Autodesk Fusion 360 part; units mm, degrees
(part 2 of 4)
sketch "Sketch8" plane through (0, 0, 1.5) normal (0, 0, 1) x (-1, 0, 0)
  line L0 (-34.7574, -85.9106) -> (-28.1106, -92.5574)
  ellipse E0 centre (-28.8177, -93.2645) end of major axis (-25.9892, -96.0929) minor radius 1 (-29.5248, -93.9716) -> (-28.1106, -92.5574) ccw
  line L1 (-29.5248, -93.9716) -> (-36.1716, -87.3248)
  ellipse E1 centre (-35.4645, -86.6177) end of major axis (-32.636, -89.4461) minor radius 1 (-34.7574, -85.9106) -> (-36.1716, -87.3248) ccw
  ellipse E2 centre (-73.5355, -93.2645) end of major axis (-70.7071, -90.436) minor radius 1 (-74.2426, -92.5574) -> (-72.8284, -93.9716) ccw
  line L2 (-74.2426, -92.5574) -> (-56.8095, -75.1242)
  ellipse E3 centre (-56.1024, -75.8313) end of major axis (-53.2739, -73.0029) minor radius 1 (-55.3953, -76.5384) -> (-56.8095, -75.1242) ccw
  line L3 (-55.3953, -76.5384) -> (-72.8284, -93.9716)
  ellipse E4 centre (-38.4645, -75.7892) end of major axis (-35.636, -78.6177) minor radius 1 (-37.7574, -75.0821) -> (-39.1716, -76.4963) ccw
  line L4 (-37.7574, -75.0821) -> (-20.2821, -92.5574)
  ellipse E5 centre (-20.9892, -93.2645) end of major axis (-18.1608, -96.0929) minor radius 1 (-21.6963, -93.9716) -> (-20.2821, -92.5574) ccw
  line L5 (-21.6963, -93.9716) -> (-39.1716, -76.4963)
  ellipse E6 centre (-58.5355, -93.9213) end of major axis (-55.7071, -91.0929) minor radius 1 (-57.5048, -94.2952) -> (-58.9094, -92.8906) ccw
  ellipse E7 centre (-57.8787, -93.2645) end of major axis (-55.0503, -90.436) minor radius 1 (-58.9094, -92.8906) -> (-57.5048, -94.2952) ccw
  ellipse E8 centre (-65.7071, -93.2645) end of major axis (-62.8787, -90.436) minor radius 1 (-66.4142, -92.5574) -> (-65, -93.9716) ccw
  line L6 (-66.4142, -92.5574) -> (-59.2426, -85.3858)
  ellipse E9 centre (-58.5355, -86.0929) end of major axis (-55.7071, -83.2645) minor radius 1 (-57.8284, -86.8) -> (-59.2426, -85.3858) ccw
  line L7 (-57.8284, -86.8) -> (-65, -93.9716)
  ellipse E10 centre (-35.6289, -93.7569) end of major axis (-32.8005, -96.5853) minor radius 1 (-35.1707, -92.8062) -> (-36.5796, -94.2151) ccw
  ellipse E11 centre (-36.1213, -93.2645) end of major axis (-33.2929, -96.0929) minor radius 1 (-36.5796, -94.2151) -> (-35.1707, -92.8062) ccw
  line L8 (-93.75, -111.8) -> (-0.25, -111.8)
  line L9 (-0.25, -111.8) -> (-0.25, -0.25)
  line L10 (-0.25, -0.25) -> (-93.75, -0.25)
  line L11 (-93.75, -0.25) -> (-93.75, -111.8)
  circle A0 centre (-5, -5) radius 2
  circle A1 centre (-3.5, -95.55) radius 2
  circle A2 centre (-90.5, -95.55) radius 2
  circle A3 centre (-87.5, -6.5) radius 2
  line L12 (-42.5, -83.8) -> (-42.5, -96.8)
  line L13 (-42.5, -96.8) -> (-51.5, -96.8)
  line L14 (-51.5, -96.8) -> (-51.5, -83.8)
  line L15 (-51.5, -83.8) -> (-42.5, -83.8)
  line L16 (-42, -100.3) -> (-42, -110.3)
  line L17 (-42, -110.3) -> (-43.9689, -110.3)
  line L18 (-43.9689, -110.3) -> (-43.9689, -103.55)
  line L19 (-43.9689, -103.55) -> (-47, -101.8)
  line L20 (-47, -101.8) -> (-50.0311, -103.55)
  line L21 (-50.0311, -103.55) -> (-50.0311, -110.3)
  line L22 (-50.0311, -110.3) -> (-52, -110.3)
  line L23 (-52, -110.3) -> (-52, -100.3)
  line L24 (-52, -100.3) -> (-55, -100.3)
  line L25 (-55, -100.3) -> (-55, -80.3)
  line L26 (-55, -80.3) -> (-52, -80.3)
  line L27 (-52, -80.3) -> (-52, -81.8)
  line L28 (-52, -81.8) -> (-53.5, -81.8)
  line L29 (-53.5, -81.8) -> (-53.5, -98.8)
  line L30 (-53.5, -98.8) -> (-40.5, -98.8)
  line L31 (-40.5, -98.8) -> (-40.5, -81.8)
  line L32 (-40.5, -81.8) -> (-42, -81.8)
  line L33 (-42, -81.8) -> (-42, -80.3)
  line L34 (-42, -80.3) -> (-39, -80.3)
  line L35 (-39, -80.3) -> (-39, -100.3)
  line L36 (-39, -100.3) -> (-42, -100.3)
  line L37 (-0.25, -111.8) -> (-15.25, -111.8)
  line L38 (-15.25, -111.8) -> (-15.25, -96.8)
  line L39 (-15.25, -96.8) -> (-0.25, -96.8)
  line L40 (-0.25, -96.8) -> (-0.25, -111.8)
  line L41 (-93.75, -0.25) -> (-78.75, -0.25)
  line L42 (-78.75, -0.25) -> (-78.75, -15.25)
  line L43 (-78.75, -15.25) -> (-93.75, -15.25)
  line L44 (-93.75, -15.25) -> (-93.75, -0.25)
  line L45 (-78.75, -15.25) -> (-15.25, -15.25)
  line L46 (-15.25, -15.25) -> (-15.25, -96.8)
  line L47 (-15.25, -96.8) -> (-78.75, -96.8)
  line L48 (-78.75, -96.8) -> (-78.75, -15.25)
  line L49 (-47, -96.8) -> (-42, -96.8)
  line L50 (-42, -96.8) -> (-42, -15.25)
  line L51 (-42, -15.25) -> (-47, -15.25)
  line L52 (-47, -15.25) -> (-47, -96.8)
  line L53 (-47, -15.25) -> (-52, -15.25)
  line L54 (-52, -15.25) -> (-52, -96.8)
  line L55 (-52, -96.8) -> (-47, -96.8)
  line L56 (-47, -96.8) -> (-47, -15.25)
  line L57 (-52, -15.25) -> (-78.75, -15.25)
  line L58 (-78.75, -15.25) -> (-78.75, -17.25)
  line L59 (-78.75, -17.25) -> (-52, -17.25)
  line L60 (-52, -17.25) -> (-52, -15.25)
  line L61 (-52, -17.25) -> (-78.75, -17.25)
  line L62 (-78.75, -17.25) -> (-78.75, -22.25)
  line L63 (-78.75, -22.25) -> (-52, -22.25)
  line L64 (-52, -22.25) -> (-52, -17.25)
  line L65 (-52, -17.25) -> (-56, -17.25)
  line L66 (-56, -17.25) -> (-56, -15.25)
  line L67 (-56, -15.25) -> (-52, -15.25)
  line L68 (-52, -15.25) -> (-52, -17.25)
  line L69 (-78.75, -17.25) -> (-74.75, -17.25)
  line L70 (-74.75, -17.25) -> (-74.75, -15.25)
  line L71 (-74.75, -15.25) -> (-78.75, -15.25)
  line L72 (-78.75, -15.25) -> (-78.75, -17.25)
  ellipse E12 centre (-56, -16.25) end of major axis (-56, -17.25) minor radius 4
  line L73 (-56, -15.25) -> (-56, -17.25)
  line L74 (-60, -16.25) -> (-52, -16.25)
  ellipse E13 centre (-74.75, -16.25) end of major axis (-74.75, -17.25) minor radius 4
  line L75 (-74.75, -15.25) -> (-74.75, -17.25)
  line L76 (-78.75, -16.25) -> (-70.75, -16.25)
  line L77 (-52, -22.25) -> (-78.75, -22.25)
  ellipse E14 centre (-74.75, -23.25) end of major axis (-74.75, -24.25) minor radius 4
  line L78 (-74.75, -22.25) -> (-74.75, -24.25)
  line L79 (-78.75, -23.25) -> (-70.75, -23.25)
  line L80 (-52, -24.25) -> (-52, -22.25)
  line L81 (-78.75, -22.25) -> (-78.75, -24.25)
  line L82 (-52, -24.25) -> (-56, -24.25)
  line L83 (-52, -22.25) -> (-52, -24.25)
  line L84 (-56, -22.25) -> (-56, -24.25) construction
  line L85 (-60, -23.25) -> (-52, -23.25) construction
  line L86 (-74.75, -22.25) -> (-78.75, -22.25)
  line L87 (-78.75, -24.25) -> (-78.75, -29.25)
  line L88 (-78.75, -22.25) -> (-78.75, -24.25)
  ellipse E15 centre (-56, -23.25) end of major axis (-56, -24.25) minor radius 4
  line L89 (-56, -22.25) -> (-56, -24.25)
  line L90 (-60, -23.25) -> (-52, -23.25)
  line L91 (-74.75, -24.25) -> (-74.75, -22.25)
  line L92 (-56, -22.25) -> (-52, -22.25)
  line L93 (-52, -29.25) -> (-52, -24.25)
  line L94 (-78.75, -24.25) -> (-74.75, -24.25)
  line L95 (-78.75, -24.25) -> (-52, -24.25)
  line L96 (-52, -24.25) -> (-78.75, -24.25)
  line L97 (-56, -24.25) -> (-56, -22.25)
  line L98 (-78.75, -29.25) -> (-52, -29.25)
  line L99 (-52, -29.25) -> (-78.75, -29.25)
  line L100 (-78.75, -31.25) -> (-52, -31.25)
  line L101 (-78.75, -38.25) -> (-52, -38.25)
  line L102 (-52, -36.25) -> (-78.75, -36.25)
  line L103 (-78.75, -43.25) -> (-52, -43.25)
  line L104 (-78.75, -36.25) -> (-52, -36.25)
  line L105 (-56, -36.25) -> (-56, -38.25) construction
  line L106 (-52, -31.25) -> (-78.75, -31.25)
  line L107 (-52, -38.25) -> (-78.75, -38.25)
  line L108 (-74.75, -29.25) -> (-78.75, -29.25)
  line L109 (-56, -36.25) -> (-52, -36.25)
  line L110 (-52, -36.25) -> (-52, -38.25)
  line L111 (-56, -29.25) -> (-56, -31.25) construction
  line L112 (-52, -38.25) -> (-52, -36.25)
  line L113 (-60, -30.25) -> (-52, -30.25) construction
  line L114 (-60, -37.25) -> (-52, -37.25) construction
  ellipse E16 centre (-56, -37.25) end of major axis (-56, -38.25) minor radius 4
  line L115 (-56, -36.25) -> (-56, -38.25)
  line L116 (-60, -37.25) -> (-52, -37.25)
  ellipse E17 centre (-74.75, -37.25) end of major axis (-74.75, -38.25) minor radius 4
  line L117 (-74.75, -36.25) -> (-74.75, -38.25)
  line L118 (-78.75, -37.25) -> (-70.75, -37.25)
  line L119 (-52, -43.25) -> (-52, -38.25)
  line L120 (-56, -36.25) -> (-56, -38.25) construction
  line L121 (-78.75, -38.25) -> (-78.75, -43.25)
  line L122 (-52, -31.25) -> (-56, -31.25)
  line L123 (-74.75, -36.25) -> (-78.75, -36.25)
  line L124 (-78.75, -29.25) -> (-78.75, -31.25)
  line L125 (-78.75, -38.25) -> (-74.75, -38.25)
  line L126 (-78.75, -36.25) -> (-78.75, -38.25)
  line L127 (-56, -29.25) -> (-52, -29.25)
  line L128 (-78.75, -31.25) -> (-78.75, -36.25)
  line L129 (-74.75, -38.25) -> (-74.75, -36.25)
  line L130 (-52, -29.25) -> (-52, -31.25)
  line L131 (-78.75, -36.25) -> (-78.75, -38.25)
  line L132 (-56, -31.25) -> (-56, -29.25)
  line L133 (-56, -38.25) -> (-56, -36.25)
  line L134 (-78.75, -29.25) -> (-78.75, -31.25)
  line L135 (-60, -37.25) -> (-52, -37.25) construction
  line L136 (-78.75, -31.25) -> (-74.75, -31.25)
  line L137 (-52, -38.25) -> (-56, -38.25)
  ellipse E18 centre (-56, -30.25) end of major axis (-56, -31.25) minor radius 4
  line L138 (-56, -29.25) -> (-56, -31.25)
  line L139 (-60, -30.25) -> (-52, -30.25)
  line L140 (-74.75, -31.25) -> (-74.75, -29.25)
  line L141 (-52, -36.25) -> (-52, -31.25)
  ellipse E19 centre (-74.75, -30.25) end of major axis (-74.75, -31.25) minor radius 4
  line L142 (-74.75, -29.25) -> (-74.75, -31.25)
  line L143 (-78.75, -30.25) -> (-70.75, -30.25)
  line L144 (-52, -31.25) -> (-52, -29.25)
  line L145 (-78.75, -66.25) -> (-52, -66.25)
  line L146 (-52, -52.25) -> (-78.75, -52.25)
  line L147 (-78.75, -58.25) -> (-70.75, -58.25) construction
  line L148 (-56, -52.25) -> (-56, -50.25)
  ellipse E20 centre (-74.75, -58.25) end of major axis (-74.75, -59.25) minor radius 4
  line L149 (-74.75, -57.25) -> (-74.75, -59.25)
  line L150 (-78.75, -58.25) -> (-70.75, -58.25)
  line L151 (-78.75, -51.25) -> (-70.75, -51.25) construction
  line L152 (-56, -50.25) -> (-56, -52.25) construction
  ellipse E21 centre (-74.75, -44.25) end of major axis (-74.75, -45.25) minor radius 4
  line L153 (-74.75, -43.25) -> (-74.75, -45.25)
  line L154 (-78.75, -44.25) -> (-70.75, -44.25)
  line L155 (-60, -58.25) -> (-52, -58.25) construction
  line L156 (-56, -43.25) -> (-56, -45.25) construction
  line L157 (-78.75, -66.25) -> (-74.75, -66.25)
  line L158 (-56, -64.25) -> (-56, -66.25) construction
  line L159 (-52, -43.25) -> (-52, -45.25)
  line L160 (-60, -44.25) -> (-52, -44.25) construction
  ellipse E22 centre (-56, -58.25) end of major axis (-56, -59.25) minor radius 4
  line L161 (-56, -57.25) -> (-56, -59.25)
  line L162 (-60, -58.25) -> (-52, -58.25)
  line L163 (-52, -52.25) -> (-52, -50.25)
  line L164 (-56, -66.25) -> (-56, -64.25)
  line L165 (-56, -57.25) -> (-56, -59.25) construction
  ellipse E23 centre (-56, -44.25) end of major axis (-56, -45.25) minor radius 4
  line L166 (-56, -43.25) -> (-56, -45.25)
  line L167 (-60, -44.25) -> (-52, -44.25)
  ellipse E24 centre (-74.75, -51.25) end of major axis (-74.75, -52.25) minor radius 4
  line L168 (-74.75, -50.25) -> (-74.75, -52.25)
  line L169 (-78.75, -51.25) -> (-70.75, -51.25)
  line L170 (-74.75, -64.25) -> (-78.75, -64.25)
  line L171 (-78.75, -57.25) -> (-78.75, -59.25)
  line L172 (-78.75, -50.25) -> (-78.75, -52.25)
  line L173 (-74.75, -50.25) -> (-78.75, -50.25)
  line L174 (-74.75, -59.25) -> (-74.75, -57.25)
  line L175 (-52, -43.25) -> (-78.75, -43.25)
  line L176 (-78.75, -43.25) -> (-78.75, -45.25)
  line L177 (-60, -65.25) -> (-52, -65.25) construction
  line L178 (-52, -64.25) -> (-52, -66.25)
  line L179 (-78.75, -64.25) -> (-78.75, -66.25)
  line L180 (-56, -64.25) -> (-56, -66.25) construction
  line L181 (-74.75, -57.25) -> (-78.75, -57.25)
  line L182 (-78.75, -65.25) -> (-70.75, -65.25) construction
  line L183 (-74.75, -43.25) -> (-78.75, -43.25)
  line L184 (-52, -66.25) -> (-52, -64.25)
  line L185 (-56, -64.25) -> (-56, -66.25) construction
  line L186 (-74.75, -64.25) -> (-74.75, -66.25) construction
  line L187 (-74.75, -52.25) -> (-74.75, -50.25)
  line L188 (-74.75, -45.25) -> (-74.75, -43.25)
  line L189 (-78.75, -59.25) -> (-78.75, -64.25)
  line L190 (-52, -59.25) -> (-52, -57.25)
  line L191 (-78.75, -52.25) -> (-74.75, -52.25)
  line L192 (-78.75, -50.25) -> (-78.75, -52.25)
  line L193 (-60, -65.25) -> (-52, -65.25) construction
  line L194 (-56, -64.25) -> (-52, -64.25)
  ellipse E25 centre (-74.75, -65.25) end of major axis (-74.75, -66.25) minor radius 4
  line L195 (-74.75, -64.25) -> (-74.75, -66.25)
  line L196 (-78.75, -65.25) -> (-70.75, -65.25)
  line L197 (-78.75, -57.25) -> (-78.75, -59.25)
  line L198 (-52, -64.25) -> (-52, -59.25)
  line L199 (-78.75, -59.25) -> (-52, -59.25)
  line L200 (-56, -59.25) -> (-56, -57.25)
  line L201 (-56, -50.25) -> (-56, -52.25) construction
  line L202 (-56, -43.25) -> (-52, -43.25)
  line L203 (-60, -51.25) -> (-52, -51.25) construction
  ellipse E26 centre (-56, -51.25) end of major axis (-56, -52.25) minor radius 4
  line L204 (-56, -50.25) -> (-56, -52.25)
  line L205 (-60, -51.25) -> (-52, -51.25)
  line L206 (-56, -50.25) -> (-52, -50.25)
  line L207 (-78.75, -45.25) -> (-52, -45.25)
  line L208 (-56, -45.25) -> (-56, -43.25)
  line L209 (-52, -59.25) -> (-78.75, -59.25)
  line L210 (-78.75, -57.25) -> (-52, -57.25)
  line L211 (-78.75, -71.25) -> (-52, -71.25)
  line L212 (-78.75, -64.25) -> (-52, -64.25)
  line L213 (-52, -64.25) -> (-78.75, -64.25)
  line L214 (-52, -66.25) -> (-78.75, -66.25)
  line L215 (-78.75, -52.25) -> (-52, -52.25)
  line L216 (-60, -51.25) -> (-52, -51.25) construction
  line L217 (-78.75, -52.25) -> (-78.75, -57.25)
  line L218 (-74.75, -66.25) -> (-74.75, -64.25)
  line L219 (-56, -57.25) -> (-52, -57.25)
  line L220 (-78.75, -50.25) -> (-52, -50.25)
  line L221 (-52, -57.25) -> (-52, -52.25)
  line L222 (-52, -57.25) -> (-78.75, -57.25)
  line L223 (-52, -50.25) -> (-78.75, -50.25)
  line L224 (-52, -52.25) -> (-56, -52.25)
  line L225 (-52, -45.25) -> (-78.75, -45.25)
  line L226 (-47, -43.25) -> (-52, -43.25)
  line L227 (-78.75, -59.25) -> (-74.75, -59.25)
  line L228 (-78.75, -43.25) -> (-78.75, -45.25)
  line L229 (-78.75, -66.25) -> (-78.75, -71.25)
  line L230 (-78.75, -45.25) -> (-78.75, -50.25)
  line L231 (-60, -65.25) -> (-52, -65.25) construction
  line L232 (-52, -71.25) -> (-52, -66.25)
  ellipse E27 centre (-56, -65.25) end of major axis (-56, -66.25) minor radius 4
  line L233 (-56, -64.25) -> (-56, -66.25)
  line L234 (-60, -65.25) -> (-52, -65.25)
  line L235 (-52, -59.25) -> (-56, -59.25)
  line L236 (-78.75, -45.25) -> (-74.75, -45.25)
  line L237 (-52, -57.25) -> (-52, -59.25)
  line L238 (-78.75, -64.25) -> (-78.75, -66.25)
  line L239 (-52, -66.25) -> (-56, -66.25)
  line L240 (-52, -45.25) -> (-56, -45.25)
  line L241 (-52, -50.25) -> (-52, -45.25)
  line L242 (-52, -45.25) -> (-52, -43.25)
  line L243 (-52, -50.25) -> (-52, -52.25)
  line L244 (-15.25, -57.25) -> (-15.25, -52.25)
  line L245 (-15.25, -24.25) -> (-42, -24.25)
  line L246 (-42, -59.25) -> (-15.25, -59.25)
  line L247 (-15.25, -66.25) -> (-42, -66.25)
  line L248 (-42, -57.25) -> (-15.25, -57.25)
  line L249 (-15.25, -64.25) -> (-42, -64.25)
  ellipse E28 centre (-19.25, -44.25) end of major axis (-19.25, -45.25) minor radius 4
  line L250 (-19.25, -43.25) -> (-19.25, -45.25)
  line L251 (-23.25, -44.25) -> (-15.25, -44.25)
  line L252 (-42, -45.25) -> (-15.25, -45.25)
  line L253 (-15.25, -50.25) -> (-42, -50.25)
  line L254 (-15.25, -36.25) -> (-42, -36.25)
  line L255 (-15.25, -52.25) -> (-42, -52.25)
  line L256 (-42, -24.25) -> (-15.25, -24.25)
  line L257 (-23.25, -51.25) -> (-15.25, -51.25) construction
  line L258 (-15.25, -29.25) -> (-42, -29.25)
  line L259 (-15.25, -38.25) -> (-42, -38.25)
  line L260 (-15.25, -64.25) -> (-15.25, -66.25)
  line L261 (-19.25, -66.25) -> (-19.25, -64.25)
  line L262 (-19.25, -43.25) -> (-15.25, -43.25)
  line L263 (-42, -22.25) -> (-15.25, -22.25)
  line L264 (-42, -29.25) -> (-15.25, -29.25)
  line L265 (-42, -59.25) -> (-42, -64.25)
  line L266 (-19.25, -50.25) -> (-15.25, -50.25)
  ellipse E29 centre (-19.25, -58.25) end of major axis (-19.25, -59.25) minor radius 4
  line L267 (-19.25, -57.25) -> (-19.25, -59.25)
  line L268 (-23.25, -58.25) -> (-15.25, -58.25)
  ellipse E30 centre (-19.25, -65.25) end of major axis (-19.25, -66.25) minor radius 4
  line L269 (-19.25, -64.25) -> (-19.25, -66.25)
  line L270 (-23.25, -65.25) -> (-15.25, -65.25)
  line L271 (-15.25, -59.25) -> (-19.25, -59.25)
  line L272 (-19.25, -50.25) -> (-19.25, -52.25) construction
  line L273 (-19.25, -15.25) -> (-19.25, -17.25) construction
  line L274 (-42, -38.25) -> (-42, -43.25)
  line L275 (-38, -24.25) -> (-38, -22.25)
  line L276 (-42, -65.25) -> (-34, -65.25) construction
  line L277 (-19.25, -24.25) -> (-19.25, -22.25)
  line L278 (-15.25, -38.25) -> (-19.25, -38.25)
  line L279 (-15.25, -22.25) -> (-15.25, -24.25)
  line L280 (-15.25, -29.25) -> (-15.25, -31.25)
  line L281 (-42, -58.25) -> (-34, -58.25) construction
  line L282 (-23.25, -30.25) -> (-15.25, -30.25) construction
  line L283 (-15.25, -24.25) -> (-19.25, -24.25)
  line L284 (-23.25, -37.25) -> (-15.25, -37.25) construction
  line L285 (-23.25, -51.25) -> (-15.25, -51.25) construction
  line L286 (-23.25, -16.25) -> (-15.25, -16.25) construction
  line L287 (-15.25, -50.25) -> (-15.25, -45.25)
  line L288 (-15.25, -31.25) -> (-15.25, -29.25)
  line L289 (-19.25, -36.25) -> (-15.25, -36.25)
  line L290 (-42, -24.25) -> (-38, -24.25)
  line L291 (-42, -31.25) -> (-38, -31.25)
  line L292 (-15.25, -38.25) -> (-15.25, -36.25)
  line L293 (-38, -59.25) -> (-38, -57.25)
  line L294 (-19.25, -29.25) -> (-19.25, -31.25) construction
  line L295 (-19.25, -50.25) -> (-19.25, -52.25) construction
  line L296 (-19.25, -36.25) -> (-19.25, -38.25) construction
  line L297 (-23.25, -23.25) -> (-15.25, -23.25) construction
  line L298 (-42, -44.25) -> (-34, -44.25) construction
  line L299 (-42, -16.25) -> (-34, -16.25) construction
  ellipse E31 centre (-19.25, -16.25) end of major axis (-19.25, -17.25) minor radius 4
  line L300 (-19.25, -15.25) -> (-19.25, -17.25)
  line L301 (-23.25, -16.25) -> (-15.25, -16.25)
  line L302 (-42, -15.25) -> (-42, -17.25)
  line L303 (-19.25, -31.25) -> (-19.25, -29.25)
  line L304 (-19.25, -45.25) -> (-19.25, -43.25)
  line L305 (-38, -22.25) -> (-42, -22.25)
  line L306 (-42, -22.25) -> (-42, -24.25)
  line L307 (-15.25, -45.25) -> (-15.25, -43.25)
  ellipse E32 centre (-38, -65.25) end of major axis (-38, -66.25) minor radius 4
  line L308 (-38, -64.25) -> (-38, -66.25)
  line L309 (-42, -65.25) -> (-34, -65.25)
  line L310 (-19.25, -36.25) -> (-19.25, -38.25) construction
  line L311 (-42, -58.25) -> (-34, -58.25) construction
  line L312 (-19.25, -50.25) -> (-19.25, -52.25) construction
  ellipse E33 centre (-38, -58.25) end of major axis (-38, -59.25) minor radius 4
  line L313 (-38, -57.25) -> (-38, -59.25)
  line L314 (-42, -58.25) -> (-34, -58.25)
  line L315 (-38, -64.25) -> (-38, -66.25) construction
  line L316 (-42, -51.25) -> (-34, -51.25) construction
  line L317 (-19.25, -15.25) -> (-15.25, -15.25)
  line L318 (-23.25, -51.25) -> (-15.25, -51.25) construction
  line L319 (-42, -15.25) -> (-42, -17.25)
  line L320 (-19.25, -38.25) -> (-19.25, -36.25)
  line L321 (-38, -22.25) -> (-38, -24.25) construction
  line L322 (-42, -22.25) -> (-42, -24.25)
  line L323 (-19.25, -17.25) -> (-19.25, -15.25)
  line L324 (-15.25, -52.25) -> (-19.25, -52.25)
  line L325 (-19.25, -29.25) -> (-15.25, -29.25)
  ellipse E34 centre (-19.25, -51.25) end of major axis (-19.25, -52.25) minor radius 4
  line L326 (-19.25, -50.25) -> (-19.25, -52.25)
  line L327 (-23.25, -51.25) -> (-15.25, -51.25)
  line L328 (-23.25, -58.25) -> (-15.25, -58.25) construction
  line L329 (-15.25, -45.25) -> (-42, -45.25)
  line L330 (-42, -31.25) -> (-42, -36.25)
  ellipse E35 centre (-38, -51.25) end of major axis (-38, -52.25) minor radius 4
  line L331 (-38, -50.25) -> (-38, -52.25)
  line L332 (-42, -51.25) -> (-34, -51.25)
  line L333 (-38, -52.25) -> (-38, -50.25)
  line L334 (-42, -45.25) -> (-42, -50.25)
  line L335 (-38, -31.25) -> (-38, -29.25)
  line L336 (-42, -52.25) -> (-38, -52.25)
  ellipse E36 centre (-38, -37.25) end of major axis (-38, -38.25) minor radius 4
  line L337 (-38, -36.25) -> (-38, -38.25)
  line L338 (-42, -37.25) -> (-34, -37.25)
  line L339 (-42, -50.25) -> (-42, -52.25)
  line L340 (-42, -38.25) -> (-38, -38.25)
  line L341 (-42, -30.25) -> (-34, -30.25) construction
  line L342 (-42, -36.25) -> (-42, -38.25)
  ellipse E37 centre (-38, -44.25) end of major axis (-38, -45.25) minor radius 4
  line L343 (-38, -43.25) -> (-38, -45.25)
  line L344 (-42, -44.25) -> (-34, -44.25)
  line L345 (-42, -43.25) -> (-42, -45.25)
  line L346 (-38, -50.25) -> (-42, -50.25)
  line L347 (-38, -43.25) -> (-42, -43.25)
  line L348 (-42, -29.25) -> (-42, -31.25)
  line L349 (-38, -38.25) -> (-38, -36.25)
  line L350 (-23.25, -23.25) -> (-15.25, -23.25) construction
  ellipse E38 centre (-38, -30.25) end of major axis (-38, -31.25) minor radius 4
  line L351 (-38, -29.25) -> (-38, -31.25)
  line L352 (-42, -30.25) -> (-34, -30.25)
  line L353 (-19.25, -22.25) -> (-15.25, -22.25)
  line L354 (-10.25, -43.25) -> (-15.25, -43.25)
  line L355 (-15.25, -36.25) -> (-15.25, -38.25)
  line L356 (-42, -50.25) -> (-42, -52.25)
  line L357 (-38, -15.25) -> (-38, -17.25) construction
  line L358 (-19.25, -29.25) -> (-19.25, -31.25) construction
  line L359 (-15.25, -31.25) -> (-19.25, -31.25)
  line L360 (-15.25, -36.25) -> (-15.25, -31.25)
  line L361 (-42, -23.25) -> (-34, -23.25) construction
  line L362 (-23.25, -37.25) -> (-15.25, -37.25) construction
  line L363 (-38, -36.25) -> (-42, -36.25)
  line L364 (-15.25, -22.25) -> (-15.25, -17.25)
  line L365 (-38, -45.25) -> (-38, -43.25)
  ellipse E39 centre (-19.25, -30.25) end of major axis (-19.25, -31.25) minor radius 4
  line L366 (-19.25, -29.25) -> (-19.25, -31.25)
  line L367 (-23.25, -30.25) -> (-15.25, -30.25)
  line L368 (-42, -36.25) -> (-42, -38.25)
  line L369 (-15.25, -43.25) -> (-15.25, -45.25)
  line L370 (-38, -17.25) -> (-38, -15.25)
  line L371 (-23.25, -37.25) -> (-15.25, -37.25) construction
  line L372 (-19.25, -22.25) -> (-19.25, -24.25) construction
  line L373 (-19.25, -22.25) -> (-19.25, -24.25) construction
  line L374 (-15.25, -24.25) -> (-15.25, -22.25)
  line L375 (-23.25, -30.25) -> (-15.25, -30.25) construction
  ellipse E40 centre (-38, -16.25) end of major axis (-38, -17.25) minor radius 4
  line L376 (-38, -15.25) -> (-38, -17.25)
  line L377 (-42, -16.25) -> (-34, -16.25)
  line L378 (-38, -15.25) -> (-42, -15.25)
  line L379 (-38, -29.25) -> (-42, -29.25)
  ellipse E41 centre (-38, -23.25) end of major axis (-38, -24.25) minor radius 4
  line L380 (-38, -22.25) -> (-38, -24.25)
  line L381 (-42, -23.25) -> (-34, -23.25)
  line L382 (-15.25, -15.25) -> (-15.25, -17.25)
  line L383 (-42, -43.25) -> (-42, -45.25)
  ellipse E42 centre (-19.25, -37.25) end of major axis (-19.25, -38.25) minor radius 4
  line L384 (-19.25, -36.25) -> (-19.25, -38.25)
  line L385 (-23.25, -37.25) -> (-15.25, -37.25)
  line L386 (-19.25, -36.25) -> (-19.25, -38.25) construction
  line L387 (-15.25, -17.25) -> (-19.25, -17.25)
  line L388 (-42, -29.25) -> (-42, -31.25)
  line L389 (-42, -45.25) -> (-38, -45.25)
  ellipse E43 centre (-19.25, -23.25) end of major axis (-19.25, -24.25) minor radius 4
  line L390 (-19.25, -22.25) -> (-19.25, -24.25)
  line L391 (-23.25, -23.25) -> (-15.25, -23.25)
  line L392 (-23.25, -65.25) -> (-15.25, -65.25) construction
  line L393 (-42, -17.25) -> (-15.25, -17.25)
  line L394 (-42, -66.25) -> (-15.25, -66.25)
  line L395 (-42, -31.25) -> (-15.25, -31.25)
  line L396 (-15.25, -31.25) -> (-42, -31.25)
  line L397 (-19.25, -52.25) -> (-19.25, -50.25)
  line L398 (-23.25, -44.25) -> (-15.25, -44.25) construction
  line L399 (-42, -50.25) -> (-15.25, -50.25)
  line L400 (-15.25, -71.25) -> (-15.25, -66.25)
  line L401 (-23.25, -65.25) -> (-15.25, -65.25) construction
  line L402 (-23.25, -65.25) -> (-15.25, -65.25) construction
  line L403 (-42, -71.25) -> (-15.25, -71.25)
  line L404 (-15.25, -15.25) -> (-42, -15.25)
  line L405 (-42, -36.25) -> (-15.25, -36.25)
  line L406 (-15.25, -50.25) -> (-15.25, -52.25)
  line L407 (-15.25, -57.25) -> (-42, -57.25)
  line L408 (-42, -52.25) -> (-42, -57.25)
  line L409 (-38, -57.25) -> (-42, -57.25)
  line L410 (-19.25, -59.25) -> (-19.25, -57.25)
  line L411 (-38, -66.25) -> (-38, -64.25)
  line L412 (-19.25, -64.25) -> (-19.25, -66.25) construction
  line L413 (-42, -64.25) -> (-42, -66.25)
  line L414 (-15.25, -52.25) -> (-15.25, -50.25)
  line L415 (-42, -57.25) -> (-42, -59.25)
  line L416 (-15.25, -59.25) -> (-15.25, -57.25)
  line L417 (-15.25, -66.25) -> (-15.25, -64.25)
  line L418 (-19.25, -57.25) -> (-19.25, -59.25) construction
  line L419 (-42, -17.25) -> (-42, -22.25)
  line L420 (-42, -57.25) -> (-42, -59.25)
  line L421 (-42, -17.25) -> (-38, -17.25)
  line L422 (-10.25, -15.25) -> (-15.25, -15.25)
  line L423 (-42, -66.25) -> (-38, -66.25)
  line L424 (-19.25, -64.25) -> (-19.25, -66.25) construction
  line L425 (-42, -52.25) -> (-15.25, -52.25)
  line L426 (-42, -43.25) -> (-15.25, -43.25)
  line L427 (-42, -24.25) -> (-42, -29.25)
  line L428 (-38, -64.25) -> (-42, -64.25)
  line L429 (-15.25, -17.25) -> (-42, -17.25)
  line L430 (-15.25, -22.25) -> (-42, -22.25)
  line L431 (-42, -38.25) -> (-15.25, -38.25)
  line L432 (-19.25, -64.25) -> (-15.25, -64.25)
  line L433 (-19.25, -64.25) -> (-19.25, -66.25) construction
  line L434 (-42, -64.25) -> (-42, -66.25)
  line L435 (-15.25, -43.25) -> (-42, -43.25)
  line L436 (-15.25, -29.25) -> (-15.25, -24.25)
  line L437 (-15.25, -66.25) -> (-19.25, -66.25)
  line L438 (-15.25, -43.25) -> (-15.25, -38.25)
  line L439 (-15.25, -57.25) -> (-15.25, -59.25)
  line L440 (-19.25, -57.25) -> (-15.25, -57.25)
  line L441 (-42, -66.25) -> (-42, -71.25)
  line L442 (-15.25, -45.25) -> (-19.25, -45.25)
  line L443 (-15.25, -17.25) -> (-15.25, -15.25)
  line L444 (-15.25, -64.25) -> (-15.25, -59.25)
  line L445 (-19.25, -43.25) -> (-19.25, -45.25) construction
  line L446 (-42, -59.25) -> (-38, -59.25)
  line L447 (-15.25, -59.25) -> (-42, -59.25)
  line L448 (-42, -64.25) -> (-15.25, -64.25)
  point P0 (-78.75, -22.25)
  point P1 (-78.75, -29.25)
  point P2 (-78.75, -36.25)
  point P3 (-78.75, -57.25)
  point P4 (-78.75, -43.25)
  point P5 (-78.75, -50.25)
  point P6 (-78.75, -64.25)
  point P7 (-42, -29.25)
  point P8 (-42, -43.25)
  point P9 (-42, -15.25)
  point P10 (-42, -57.25)
  point P11 (-42, -22.25)
  point P12 (-42, -50.25)
  point P13 (-42, -64.25)
  point P14 (-42, -36.25)
  dimension "d133" = 15
  dimension "d134" = 15
  dimension "d135" = 15
  dimension "d136" = 15
  dimension "d137" = 5
  dimension "d138" = 5
  dimension "d148" = 2
  dimension "d149" = 5
  dimension "d150" = 4
  dimension "d151" = 4
  dimension "d152" = 2
  dimension "d153" = 5
  dimension "d154" = 4
  dimension "d155" = 4
  dimension "d156" = 2
  dimension "d157" = 5
  dimension "d158" = 4
  dimension "d159" = 4
  dimension "d160" = 2
  dimension "d161" = 5
  dimension "d162" = 4
  dimension "d163" = 4
  dimension "d164" = 5
  dimension "d165" = 2
  dimension "d166" = 5
  dimension "d167" = 4
  dimension "d168" = 4
  dimension "d169" = 2
  dimension "d170" = 5
  dimension "d171" = 4
  dimension "d172" = 4
  dimension "d173" = 2
  dimension "d174" = 5
  dimension "d175" = 4
  dimension "d176" = 4
  dimension "d177" = 2
  dimension "d178" = 5
  dimension "d179" = 4
  dimension "d180" = 4
  dimension "d181" = 5
  dimension "d182" = 2
  dimension "d183" = 5
  dimension "d184" = 4
  dimension "d185" = 4
  dimension "d186" = 2
  dimension "d187" = 5
  dimension "d188" = 4
  dimension "d189" = 4
  dimension "d190" = 2
  dimension "d191" = 5
  dimension "d192" = 4
  dimension "d193" = 4
  dimension "d194" = 2
  dimension "d195" = 5
  dimension "d196" = 4
  dimension "d197" = 4
  dimension "d198" = 5
  dimension "d199" = 2
  dimension "d200" = 5
  dimension "d201" = 4
  dimension "d202" = 4
  dimension "d203" = 2
  dimension "d204" = 5
  dimension "d205" = 4
  dimension "d206" = 4
  dimension "d207" = 2
  dimension "d208" = 5
  dimension "d209" = 4
  dimension "d210" = 4
  dimension "d211" = 2
  dimension "d212" = 5
  dimension "d213" = 4
  dimension "d214" = 4
  constraint horizontal L37
  constraint vertical L38
  constraint horizontal L39
  constraint vertical L40
  constraint coincident L8.end L9.start
  constraint horizontal L41
  constraint vertical L42
  constraint horizontal L43
  constraint vertical L44
  constraint coincident L10.end L11.start
  constraint horizontal L45
  constraint vertical L46
  constraint horizontal L47
  constraint vertical L48
  constraint horizontal L49
  constraint vertical L50
  constraint horizontal L51
  constraint vertical L52
  constraint coincident L45 P9
  constraint midpoint L13 L49.start
  constraint horizontal L53
  constraint vertical L54
  constraint horizontal L55
  constraint vertical L56
  constraint horizontal L57
  constraint vertical L58
  constraint horizontal L59
  constraint vertical L60
  constraint horizontal L61
  constraint vertical L62
  constraint horizontal L63
  constraint vertical L64
  constraint horizontal L65
  constraint vertical L66
  constraint horizontal L67
  constraint vertical L68
  constraint horizontal L69
  constraint vertical L70
  constraint horizontal L71
  constraint vertical L72
  constraint midpoint L66 E12.centre
  constraint coincident L66.end E12
  constraint coincident E12 L74.start
  constraint coincident E12 L74.end
  constraint midpoint L70 E13.centre
  constraint coincident L70.end E13
  constraint coincident E13 L76.start
  constraint coincident E13 L76.end
  constraint horizontal L77
  constraint vertical L88
  constraint horizontal L95
  constraint vertical L80
  constraint horizontal L96
  constraint vertical L87
  constraint horizontal L98
  constraint vertical L93
  constraint horizontal L82
  constraint vertical L97
  constraint horizontal L92
  constraint vertical L83
  constraint horizontal L94
  constraint vertical L91
  constraint horizontal L86
  constraint vertical L81
  constraint midpoint E15.centre L97
  constraint coincident L84.start E15
  constraint coincident L85.start E15
  constraint coincident L85.end E15
  constraint midpoint E14.centre L91
  constraint coincident L78.start E14
  constraint coincident L79.start E14
  constraint coincident L79.end E14
  constraint horizontal L99
  constraint vertical L124
  constraint horizontal L100
  constraint vertical L144
  constraint horizontal L106
  constraint vertical L128
  constraint horizontal L104
  constraint vertical L141
  constraint horizontal L122
  constraint vertical L132
  constraint horizontal L127
  constraint vertical L130
  constraint horizontal L136
  constraint vertical L140
  constraint horizontal L108
  constraint vertical L134
  constraint midpoint E18.centre L132
  constraint coincident L111.start E18
  constraint coincident L113.start E18
  constraint coincident L113.end E18
  constraint midpoint E19.centre L140
  constraint coincident L108.start E19
  constraint coincident L143.start E19
  constraint coincident L143.end E19
  constraint horizontal L102
  constraint vertical L126
  constraint horizontal L101
  constraint vertical L112
  constraint horizontal L107
  constraint vertical L121
  constraint horizontal L103
  constraint vertical L119
  constraint horizontal L137
  constraint vertical L133
  constraint horizontal L109
  constraint vertical L110
  constraint horizontal L125
  constraint vertical L129
  constraint horizontal L123
  constraint vertical L131
  constraint midpoint E16.centre L133
  constraint coincident L105.start E16
  constraint coincident L114.start E16
  constraint coincident L114.end E16
  constraint midpoint E17.centre L129
  constraint coincident L117.start E17
  constraint coincident L118.start E17
  constraint coincident L118.end E17
  constraint horizontal L226
  constraint horizontal L175
  constraint vertical L176
  constraint horizontal L207
  constraint vertical L242
  constraint horizontal L225
  constraint vertical L230
  constraint horizontal L220
  constraint vertical L241
  constraint horizontal L240
  constraint vertical L208
  constraint horizontal L202
  constraint vertical L159
  constraint horizontal L236
  constraint vertical L188
  constraint horizontal L183
  constraint vertical L228
  constraint midpoint E23.centre L208
  constraint coincident L156.start E23
  constraint coincident L160.start E23
  constraint coincident L160.end E23
  constraint midpoint E21.centre L188
  constraint coincident L153.start E21
  constraint coincident L154.start E21
  constraint coincident L154.end E21
  constraint horizontal L223
  constraint vertical L172
  constraint horizontal L215
  constraint vertical L163
  constraint horizontal L146
  constraint vertical L217
  constraint horizontal L210
  constraint vertical L221
  constraint horizontal L224
  constraint vertical L148
  constraint horizontal L206
  constraint vertical L243
  constraint horizontal L191
  constraint vertical L187
  constraint horizontal L173
  constraint vertical L192
  constraint midpoint E26.centre L148
  constraint coincident L148.end E26
  constraint coincident L203.start E26
  constraint coincident L203.end E26
  constraint midpoint E24.centre L187
  constraint coincident L168.start E24
  constraint coincident L151.start E24
  constraint coincident L151.end E24
  constraint horizontal L222
  constraint vertical L197
  constraint horizontal L199
  constraint vertical L190
  constraint horizontal L209
  constraint vertical L189
  constraint horizontal L212
  constraint vertical L198
  constraint horizontal L235
  constraint vertical L200
  constraint horizontal L219
  constraint vertical L237
  constraint horizontal L227
  constraint vertical L174
  constraint horizontal L181
  constraint vertical L171
  constraint midpoint E22.centre L200
  constraint coincident L161.start E22
  constraint coincident L155.start E22
  constraint coincident L155.end E22
  constraint midpoint E20.centre L174
  constraint coincident L149.start E20
  constraint coincident L147.start E20
  constraint coincident L147.end E20
  constraint horizontal L213
  constraint vertical L179
  constraint horizontal L145
  constraint vertical L184
  constraint horizontal L214
  constraint vertical L229
  constraint horizontal L211
  constraint vertical L232
  constraint horizontal L239
  constraint vertical L164
  constraint horizontal L194
  constraint vertical L178
  constraint horizontal L157
  constraint vertical L218
  constraint horizontal L170
  constraint vertical L238
  constraint midpoint E27.centre L164
  constraint coincident L158.start E27
  constraint coincident L177.start E27
  constraint coincident L177.end E27
  constraint midpoint E25.centre L218
  constraint coincident L170.start E25
  constraint coincident L182.start E25
  constraint coincident L182.end E25
  constraint horizontal L422
  constraint horizontal L404
  constraint vertical L319
  constraint horizontal L393
  constraint vertical L443
  constraint horizontal L429
  constraint vertical L419
  constraint horizontal L263
  constraint vertical L364
  constraint horizontal L387
  constraint vertical L323
  constraint horizontal L317
  constraint vertical L382
  constraint horizontal L421
  constraint vertical L370
  constraint horizontal L378
  constraint vertical L302
  constraint midpoint E31.centre L323
  constraint coincident L273.start E31
  constraint coincident L286.start E31
  constraint coincident L286.end E31
  constraint midpoint E40.centre L370
  constraint coincident L357.start E40
  constraint coincident L299.start E40
  constraint coincident L299.end E40
  constraint horizontal L430
  constraint vertical L306
  constraint horizontal L256
  constraint vertical L374
  constraint horizontal L245
  constraint vertical L427
  constraint horizontal L264
  constraint vertical L436
  constraint horizontal L283
  constraint vertical L277
  constraint horizontal L353
  constraint vertical L279
  constraint horizontal L290
  constraint vertical L275
  constraint horizontal L305
  constraint vertical L322
  constraint midpoint E43.centre L277
  constraint coincident L277.end E43
  constraint coincident L297.start E43
  constraint coincident L297.end E43
  constraint midpoint E41.centre L275
  constraint coincident L275.end E41
  constraint coincident L361.start E41
  constraint coincident L361.end E41
  constraint horizontal L258
  constraint vertical L388
  constraint horizontal L395
  constraint vertical L288
  constraint horizontal L396
  constraint vertical L330
  constraint horizontal L405
  constraint vertical L360
  constraint horizontal L359
  constraint vertical L303
  constraint horizontal L325
  constraint vertical L280
  constraint horizontal L291
  constraint vertical L335
  constraint horizontal L379
  constraint vertical L348
  constraint midpoint E39.centre L303
  constraint coincident L294.start E39
  constraint coincident L282.start E39
  constraint coincident L282.end E39
  constraint midpoint E38.centre L335
  constraint coincident L335.end E38
  constraint coincident L341.start E38
  constraint coincident L341.end E38
  constraint horizontal L254
  constraint vertical L342
  constraint horizontal L431
  constraint vertical L292
  constraint horizontal L259
  constraint vertical L274
  constraint horizontal L426
  constraint vertical L438
  constraint horizontal L278
  constraint vertical L320
  constraint horizontal L289
  constraint vertical L355
  constraint horizontal L340
  constraint vertical L349
  constraint horizontal L363
  constraint vertical L368
  constraint midpoint E42.centre L320
  constraint coincident L289.start E42
  constraint coincident L284.start E42
  constraint coincident L284.end E42
  constraint midpoint E36.centre L349
  constraint coincident L337.start E36
  constraint coincident L338.start E36
  constraint coincident L338.end E36
  constraint horizontal L354
  constraint horizontal L435
  constraint vertical L383
  constraint horizontal L252
  constraint vertical L307
  constraint horizontal L329
  constraint vertical L334
  constraint horizontal L399
  constraint vertical L287
  constraint horizontal L442
  constraint vertical L304
  constraint horizontal L262
  constraint vertical L369
  constraint horizontal L389
  constraint vertical L365
  constraint horizontal L347
  constraint vertical L345
  constraint midpoint E28.centre L304
  constraint coincident L250.start E28
  constraint coincident L251.start E28
  constraint coincident L251.end E28
  constraint midpoint E37.centre L365
  constraint coincident L343.start E37
  constraint coincident L298.start E37
  constraint coincident L298.end E37
  constraint horizontal L253
  constraint vertical L356
  constraint horizontal L425
  constraint vertical L414
  constraint horizontal L255
  constraint vertical L408
  constraint horizontal L248
  constraint vertical L244
  constraint horizontal L324
  constraint vertical L397
  constraint horizontal L266
  constraint vertical L406
  constraint horizontal L336
  constraint vertical L333
  constraint horizontal L346
  constraint vertical L339
  constraint midpoint E34.centre L397
  constraint coincident L266.start E34
  constraint coincident L257.start E34
  constraint coincident L257.end E34
  constraint midpoint E35.centre L333
  constraint coincident L331.start E35
  constraint coincident L316.start E35
  constraint coincident L316.end E35
  constraint horizontal L407
  constraint vertical L420
  constraint horizontal L246
  constraint vertical L416
  constraint horizontal L447
  constraint vertical L265
  constraint horizontal L448
  constraint vertical L444
  constraint horizontal L271
  constraint vertical L410
  constraint horizontal L440
  constraint vertical L439
  constraint horizontal L446
  constraint vertical L293
  constraint horizontal L409
  constraint vertical L415
  constraint midpoint E29.centre L410
  constraint coincident L267.start E29
  constraint coincident L268.start E29
  constraint coincident L268.end E29
  constraint midpoint E33.centre L293
  constraint coincident L293.end E33
  constraint coincident L281.start E33
  constraint coincident L281.end E33
  constraint horizontal L249
  constraint vertical L434
  constraint horizontal L394
  constraint vertical L417
  constraint horizontal L247
  constraint vertical L441
  constraint horizontal L403
  constraint vertical L400
  constraint horizontal L437
  constraint vertical L261
  constraint horizontal L432
  constraint vertical L260
  constraint horizontal L423
  constraint vertical L411
  constraint horizontal L428
  constraint vertical L413
  constraint midpoint E30.centre L261
  constraint coincident L261.end E30
  constraint coincident L270.start E30
  constraint coincident L270.end E30
  constraint midpoint E32.centre L411
  constraint coincident L308.start E32
  constraint coincident L276.start E32
  constraint coincident L276.end E32
  measures "d133" distance of L8.end L37.end
  measures "d134" distance of L8.end L39.end
  measures "d135" distance of L10.end L41.end
  measures "d136" distance of L10.end L43.end
  measures "d137" distance of L49.start L49.end
  measures "d138" distance of L51.end L53.end
  measures "d148" distance of L53.end L59.end
  measures "d149" distance of L59.end L63.end
  measures "d150" distance of L59.end L65.end
  measures "d151" distance of L58.end L69.end
  measures "d152" distance of L63.end L80.start
  measures "d153" distance of L93.start L80.start
  measures "d154" distance of L80.start L82.end
  measures "d155" distance of L81.end L78.end
  measures "d156" distance of L93.start L100.end
  measures "d157" distance of L102.start L100.end
  measures "d158" distance of L100.end L111.end
  measures "d159" distance of L100.start L136.end
  measures "d160" distance of L102.start L101.end
  measures "d161" distance of L103.end L101.end
  measures "d162" distance of L105.end L101.end
  measures "d163" distance of L117.end L101.start
  measures "d164" distance of L103.end L226.start
  measures "d165" distance of L103.end L159.end
  measures "d166" distance of L163.end L159.end
  measures "d167" distance of L159.end L156.end
  measures "d168" distance of L176.end L153.end
  measures "d169" distance of L163.end L146.start
  measures "d170" distance of L190.end L146.start
  measures "d171" distance of L148.start L146.start
  measures "d172" distance of L168.end L146.end
  measures "d173" distance of L190.start L190.end
  measures "d174" distance of L190.start L178.start
  measures "d175" distance of L190.start L161.end
  measures "d176" distance of L171.end L149.end
  measures "d177" distance of L178.start L145.end
  measures "d178" distance of L211.end L145.end
  measures "d179" distance of L158.end L145.end
  measures "d180" distance of L157.end L145.start
  measures "d181" distance of L45.end L422.start
  measures "d182" distance of L45.end L364.end
  measures "d183" distance of L263.end L364.end
  measures "d184" distance of L364.end L273.end
  measures "d185" distance of L302.end L357.end
  measures "d186" distance of L263.end L245.start
  measures "d187" distance of L258.start L245.start
  measures "d188" distance of L277.start L245.start
  measures "d189" distance of L275.start L245.end
  measures "d190" distance of L280.end L258.start
  measures "d191" distance of L280.end L254.start
  measures "d192" distance of L280.end L294.end
  measures "d193" distance of L291.start L291.end
  measures "d194" distance of L254.start L259.start
  measures "d195" distance of L262.end L259.start
  measures "d196" distance of L278.end L259.start
  measures "d197" distance of L337.end L259.end
  measures "d198" distance of L262.end L354.start
  measures "d199" distance of L252.end L262.end
  measures "d200" distance of L252.end L253.start
  measures "d201" distance of L252.end L250.end
  measures "d202" distance of L252.start L343.end
  measures "d203" distance of L253.start L244.end
  measures "d204" distance of L244.start L244.end
  measures "d205" distance of L272.end L244.end
  measures "d206" distance of L331.end L255.end
  measures "d207" distance of L246.end L244.start
  measures "d208" distance of L246.end L249.start
  measures "d209" distance of L246.end L267.end
  measures "d210" distance of L246.start L293.start
  measures "d211" distance of L249.start L247.start
  measures "d212" distance of L247.start L400.start
  measures "d213" distance of L247.start L261.start
  measures "d214" distance of L308.end L247.end
extrude "Extrude12" cut sketch "Sketch8" against normal blind 11 contours L70 E13 L75 L76 | L45 L57 L59 L61 E12 E13 | L70 E13 L75 L76 | L70 E13 L75 L76 | L66 E12 L73 L74 | L66 E12 L73 L74 | L70 E13 L75 L76 | L261 E30 L269 L270 | L261 E30 L269 L270 | L261 E30 L269 L270 | L247 L249 E30 E32 L394 L448 | L66 E12 L73 L74 | L66 E12 L73 L74 | L261 E30 L269 L270 | E32 L308 L309 L411 | E32 L308 L309 L411 | E32 L308 L309 L411 | E14 L78 L79 L91 | E14 L78 L79 L91 | L63 L77 E14 E15 L95 L96 | E14 L78 L79 L91 | E32 L308 L309 L411 | E14 L78 L79 L91 | E15 L89 L90 L97 | E15 L89 L90 L97 | E29 L267 L268 L410 | E29 L267 L268 L410 | L246 L248 E29 E33 L407 L447 | E29 L267 L268 L410 | L370 E40 L376 L377 | L45 E31 E40 L393 L404 L429 | L370 E40 L376 L377 | L370 E40 L376 L377 | E15 L89 L90 L97 | E15 L89 L90 L97 | E29 L267 L268 L410 | L293 E33 L313 L314 | L293 E33 L313 L314 | L293 E33 L313 L314 | E31 L300 L301 L323 | E31 L300 L301 L323 | L370 E40 L376 L377 | E23 L166 L167 L208 | E23 L166 L167 L208 | L103 E21 E23 L175 L207 L225 | E23 L166 L167 L208 | L140 E19 L142 L143 | L140 E19 L142 L143 | L140 E19 L142 L143 | L98 L99 L100 L106 E18 E19 | L293 E33 L313 L314 | E31 L300 L301 L323 | E31 L300 L301 L323 | E16 L115 L116 L133 | E16 L115 L116 L133 | L101 L102 L104 L107 E16 E17 | E16 L115 L116 L133 | E23 L166 L167 L208 | E21 L153 L154 L188 | E21 L153 L154 L188 | L140 E19 L142 L143 | L132 E18 L138 L139 | L132 E18 L138 L139 | E34 L326 L327 L397 | E34 L326 L327 L397 | L253 L255 E34 E35 L399 L425 | E34 L326 L327 L397 | L275 E41 L380 L381 | L275 E41 L380 L381 | L275 E41 L380 L381 | L245 L256 L263 E41 E43 L430 | E16 L115 L116 L133 | E17 L117 L118 L129 | E17 L117 L118 L129 | E21 L153 L154 L188 | E21 L153 L154 L188 | L132 E18 L138 L139 | L132 E18 L138 L139 | E34 L326 L327 L397 | E35 L331 L332 L333 | E35 L331 L332 L333 | E35 L331 L332 L333 | E25 L195 L196 L218 | E25 L195 L196 L218 | L145 E25 L212 L213 L214 E27 | E25 L195 L196 L218 | L275 E41 L380 L381 | L277 E43 L390 L391 | L277 E43 L390 L391 | E17 L117 L118 L129 | E17 L117 L118 L129 | L148 E26 L204 L205 | L148 E26 L204 L205 | L148 E26 L204 L205 | L146 E24 E26 L215 L220 L223 | E35 L331 L332 L333 | L164 E27 L233 L234 | L164 E27 L233 L234 | L164 E27 L233 L234 | E25 L195 L196 L218 | L277 E43 L390 L391 | L277 E43 L390 L391 | L148 E26 L204 L205 | E24 L168 L169 L187 | E24 L168 L169 L187 | E28 L250 L251 L304 | E28 L250 L251 L304 | E28 L252 L329 E37 L426 L435 | E28 L250 L251 L304 | L164 E27 L233 L234 | L335 E38 L351 L352 | L335 E38 L351 L352 | L335 E38 L351 L352 | L258 L264 E38 E39 L395 L396 | E24 L168 L169 L187 | E24 L168 L169 L187 | E28 L250 L251 L304 | E37 L343 L344 L365 | E37 L343 L344 L365 | E37 L343 L344 L365 | E20 L149 L150 L174 | E20 L149 L150 L174 | E20 L149 L150 L174 | E20 E22 L199 L209 L210 L222 | L335 E38 L351 L352 | L303 E39 L366 L367 | L303 E39 L366 L367 | E22 L161 L162 L200 | E22 L161 L162 L200 | E22 L161 L162 L200 | E37 L343 L344 L365 | E22 L161 L162 L200 | E20 L149 L150 L174 | L303 E39 L366 L367 | L303 E39 L366 L367 | L320 E42 L384 L385 | L320 E42 L384 L385 | L320 E42 L384 L385 | L254 L259 E36 E42 L405 L431 | E36 L337 L338 L349 | E36 L337 L338 L349 | E36 L337 L338 L349 | L320 E42 L384 L385 | E36 L337 L338 L349